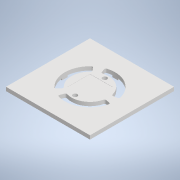
# Autodesk Inventor part: CubeFace
Saved by Autodesk Inventor 2022 (Build 260153000, 153)
## iProperties
Created: 2022-04-08
Part Number: CubeFace
Material: Generic
Document SubType Name: Modeling
Designer: awp
Density: 1 g/cm^3
Appearance: Default
Author: awp
Autodesk Inventor part; units mm, degrees
ref_plane "YZ Plane" through (0, 0, 0) normal (1, 0, 0) x (0, 1, 0)
ref_plane "XZ Plane" through (0, 0, 0) normal (0, 1, 0) x (-1, 0, 0)
ref_plane "XY Plane" through (0, 0, 0) normal (0, 0, 1) x (1, 0, 0)
sketch "Sketch1" plane through (0, 0, 0) normal (0, 1, 0) x (-1, 0, 0)
  line L0 (0, 0) -> (57.5, 0)
  line L1 (57.5, 0) -> (57.5, -57.5)
  line L2 (57.5, -57.5) -> (0, -57.5)
  line L3 (0, -57.5) -> (0, 0)
  dimension "d0" = 57.5
  dimension "d1" = 57.5
  constraints: 8 end point, 2 parallel, 1 horizontal, 1 perpendicular
  measures "d0" distance of L1.end L2.end
  measures "d1" distance of L0.end L1.end
extrude "Extrusion1" add sketch "Sketch1" along normal blind 2.54
sketch "Sketch2" plane through (0, 0, 0) normal (0, -1, 0) x (1, 0, 0)
  line L0 (0, -57.5) -> (-57.5, -57.5) projected
  line L1 (0, 0) -> (0, -57.5) projected
  line L2 (-57.5, 0) -> (0, 0) projected
  line L3 (-57.5, -57.5) -> (-57.5, 0) projected
  line L4 (-57.5, -57.5) -> (-57.5, 0) projected
  line L5 (-57.5, -57.5) -> (-38.3333, -57.5)
  line L6 (-38.3333, -57.5) -> (-38.3333, -38.3333)
  line L7 (-38.3333, -38.3333) -> (-57.5, -38.3333)
  line L8 (-57.5, -38.3333) -> (-57.5, -57.5)
  line L9 (-57.5, -38.3333) -> (-38.3333, -38.3333)
  line L10 (-38.3333, -38.3333) -> (-38.3333, -19.1667)
  line L11 (-38.3333, -19.1667) -> (-57.5, -19.1667)
  line L12 (-57.5, -19.1667) -> (-57.5, -38.3333)
  line L13 (-57.5, 0) -> (0, 0) projected
  line L14 (-57.5, -19.1667) -> (-38.3333, -19.1667)
  line L15 (-38.3333, -19.1667) -> (-38.3333, 0)
  line L16 (-38.3333, 0) -> (-57.5, 0)
  line L17 (-57.5, 0) -> (-57.5, -19.1667)
  line L18 (-38.3333, 0) -> (-19.1667, 0)
  line L19 (-19.1667, 0) -> (-19.1667, -19.1667)
  line L20 (-19.1667, -19.1667) -> (-38.3333, -19.1667)
  line L21 (-38.3333, -19.1667) -> (-38.3333, 0)
  line L22 (-19.1667, -19.1667) -> (0, -19.1667)
  line L23 (0, -19.1667) -> (0, 0)
  line L24 (0, 0) -> (-19.1667, 0)
  line L25 (-19.1667, 0) -> (-19.1667, -19.1667)
  line L26 (-19.1667, -19.1667) -> (-38.3333, -19.1667)
  line L27 (-38.3333, -19.1667) -> (-38.3333, -38.3333)
  line L28 (-38.3333, -38.3333) -> (-19.1667, -38.3333)
  line L29 (-19.1667, -38.3333) -> (-19.1667, -19.1667)
  line L30 (-19.1667, -38.3333) -> (-38.3333, -38.3333)
  line L31 (-38.3333, -38.3333) -> (-38.3333, -57.5)
  line L32 (-38.3333, -57.5) -> (-19.1667, -57.5)
  line L33 (-19.1667, -57.5) -> (-19.1667, -38.3333)
  line L34 (0, -19.1667) -> (-19.1667, -19.1667)
  line L35 (-19.1667, -19.1667) -> (-19.1667, -38.3333)
  line L36 (-19.1667, -38.3333) -> (0, -38.3333)
  line L37 (0, -38.3333) -> (0, -19.1667)
  line L38 (0, -38.3333) -> (-19.1667, -38.3333)
  line L39 (-19.1667, -38.3333) -> (-19.1667, -57.5)
  line L40 (-19.1667, -57.5) -> (0, -57.5)
  line L41 (0, -57.5) -> (0, -38.3333)
  line L42 (0, -57.5) -> (-57.5, -57.5) projected
  line L43 (-57.5, -57.5) -> (-56.23, -57.5)
  line L44 (-56.23, -57.5) -> (-56.23, -56.23)
  line L45 (-56.23, -56.23) -> (-57.5, -56.23)
  line L46 (-57.5, -56.23) -> (-57.5, -57.5)
  line L47 (-38.3333, -38.3333) -> (-52.3033, -38.3333)
  line L48 (-52.3033, -38.3333) -> (-52.3033, -52.3033)
  line L49 (-52.3033, -52.3033) -> (-38.3333, -52.3033)
  line L50 (-38.3333, -52.3033) -> (-38.3333, -38.3333)
  line L51 (-52.3033, -52.3033) -> (-56.23, -52.3033)
  line L52 (-56.23, -52.3033) -> (-56.23, -56.23)
  line L53 (-56.23, -56.23) -> (-52.3033, -56.23)
  line L54 (-52.3033, -56.23) -> (-52.3033, -52.3033)
  line L55 (-56.23, -26.7867) -> (-56.23, -30.7133)
  line L56 (-56.23, -30.7133) -> (-52.3033, -30.7133)
  line L57 (-52.3033, -26.7867) -> (-56.23, -26.7867)
  line L58 (-52.3033, -30.7133) -> (-52.3033, -26.7867)
  line L59 (-56.23, -1.27) -> (-56.23, -5.1967)
  line L60 (-56.23, -5.1967) -> (-52.3033, -5.1967)
  line L61 (-52.3033, -1.27) -> (-56.23, -1.27)
  line L62 (-52.3033, -5.1967) -> (-52.3033, -1.27)
  line L63 (-30.7133, -52.3033) -> (-30.7133, -56.23)
  line L64 (-30.7133, -56.23) -> (-26.7867, -56.23)
  line L65 (-26.7867, -52.3033) -> (-30.7133, -52.3033)
  line L66 (-26.7867, -56.23) -> (-26.7867, -52.3033)
  line L67 (-30.7133, -26.7867) -> (-30.7133, -30.7133)
  line L68 (-30.7133, -30.7133) -> (-26.7867, -30.7133)
  line L69 (-26.7867, -26.7867) -> (-30.7133, -26.7867)
  line L70 (-26.7867, -30.7133) -> (-26.7867, -26.7867)
  line L71 (-30.7133, -1.27) -> (-30.7133, -5.1967)
  line L72 (-30.7133, -5.1967) -> (-26.7867, -5.1967)
  line L73 (-26.7867, -1.27) -> (-30.7133, -1.27)
  line L74 (-26.7867, -5.1967) -> (-26.7867, -1.27)
  line L75 (-5.1967, -52.3033) -> (-5.1967, -56.23)
  line L76 (-5.1967, -56.23) -> (-1.27, -56.23)
  line L77 (-1.27, -52.3033) -> (-5.1967, -52.3033)
  line L78 (-1.27, -56.23) -> (-1.27, -52.3033)
  line L79 (-5.1967, -26.7867) -> (-5.1967, -30.7133)
  line L80 (-5.1967, -30.7133) -> (-1.27, -30.7133)
  line L81 (-1.27, -26.7867) -> (-5.1967, -26.7867)
  line L82 (-1.27, -30.7133) -> (-1.27, -26.7867)
  line L83 (-5.1967, -1.27) -> (-5.1967, -5.1967)
  line L84 (-5.1967, -5.1967) -> (-1.27, -5.1967)
  line L85 (-1.27, -1.27) -> (-5.1967, -1.27)
  line L86 (-1.27, -5.1967) -> (-1.27, -1.27)
  dimension "d5" = 19.1667
  dimension "d6" = 19.1667
  dimension "d7" = 19.1667
  dimension "d8" = 19.1667
  dimension "d9" = 1.27
  dimension "d10" = 1.27
  dimension "d11" = 13.97
  dimension "d12" = 13.97
  dimension "d15" = 25.5167
  dimension "d18" = 25.5167
  constraints: 160 end point, 24 parallel, 13 horizontal, 12 perpendicular, 2 collinear, 2 point on line, 1 vertical, 62 other
  measures "d5" distance of L5.end L6.end
  measures "d6" distance of L10.end L11.end
  measures "d7" distance of L9.end L10.end
  measures "d8" distance of L19.end L20.end
  measures "d9" distance of L45.end L44.end
  measures "d10" distance of L44.end L43.end
  measures "d11" distance of L49.end L48.end
  measures "d12" distance of L48.end L47.end
  measures "d15" distance of L51.end L55.start
  measures "d18" distance of L51.end L63.start
extrude "Extrusion2" add sketch "Sketch2" along normal blind 1.27 contours L52 L51 L54 L53 | L57 L58 L56 L55 | L61 L62 L60 L59 | L65 L66 L64 L63 | L69 L70 L68 L67 | L73 L74 L72 L71 | L77 L78 L76 L75 | L81 L82 L80 L79 | L85 L86 L84 L83
chamfer "Chamfer1" [suppressed]
sketch "Sketch3" plane through (0, 2.54, 0) normal (0, 1, 0) x (1, 0, 0)
  line L0 (0, 57.5) -> (-57.5, 57.5) projected
  line L1 (-57.5, 57.5) -> (-57.5, 0) projected
  line L2 (-57.5, 0) -> (0, 0) projected
  line L3 (0, 0) -> (0, 57.5) projected
  line L4 (-28.75, 28.75) -> (-36.37, 28.75)
  line L5 (-36.37, 28.75) -> (-36.37, 21.13)
  line L6 (-36.37, 21.13) -> (-28.75, 21.13)
  line L7 (-28.75, 21.13) -> (-28.75, 28.75)
  line L8 (-36.37, 21.13) -> (-21.13, 21.13)
  line L9 (-21.13, 21.13) -> (-21.13, 36.37)
  line L10 (-21.13, 36.37) -> (-36.37, 36.37)
  line L11 (-36.37, 36.37) -> (-36.37, 21.13)
  dimension "d26" = 7.62
  dimension "d27" = 7.62
  dimension "d30" = 15.24
  dimension "d31" = 15.24
  constraints: 16 end point, 4 parallel, 2 horizontal, 2 perpendicular
  measures "d26" distance of L6.end L5.end
  measures "d27" distance of L5.end L4.end
  measures "d30" distance of L10.end L9.end
  measures "d31" distance of L9.end L8.end
extrude "Extrusion3" cut sketch "Sketch3" against normal blind 0.127 contours L7 L6 L5 L4 | L4 L11 L10 L9 L8 L7
sketch "Sketch4" plane through (0, 0, 0) normal (0, -1, 0) x (1, 0, 0)
  line L0 (-56.23, -5.1967) -> (-56.23, -1.27) projected
  line L1 (-56.23, -1.27) -> (-52.3033, -1.27) projected
  line L2 (-52.3033, -1.27) -> (-52.3033, -5.1967) projected
  line L3 (-30.7133, -56.23) -> (-30.7133, -52.3033) projected
  line L4 (-30.7133, -52.3033) -> (-26.7867, -52.3033) projected
  line L5 (-26.7867, -52.3033) -> (-26.7867, -56.23) projected
  line L6 (-26.7867, -56.23) -> (-30.7133, -56.23) projected
  line L7 (-5.1967, -5.1967) -> (-5.1967, -1.27) projected
  line L8 (-5.1967, -1.27) -> (-1.27, -1.27) projected
  line L9 (-1.27, -1.27) -> (-1.27, -5.1967) projected
  line L10 (-1.27, -5.1967) -> (-5.1967, -5.1967) projected
  line L11 (-5.1967, -30.7133) -> (-5.1967, -26.7867) projected
  line L12 (-5.1967, -26.7867) -> (-1.27, -26.7867) projected
  line L13 (-1.27, -26.7867) -> (-1.27, -30.7133) projected
  line L14 (-1.27, -30.7133) -> (-5.1967, -30.7133) projected
  line L15 (-30.7133, -30.7133) -> (-30.7133, -26.7867) projected
  line L16 (-30.7133, -26.7867) -> (-26.7867, -26.7867) projected
  line L17 (-26.7867, -26.7867) -> (-26.7867, -30.7133) projected
  line L18 (-26.7867, -30.7133) -> (-30.7133, -30.7133) projected
  line L19 (-56.23, -30.7133) -> (-56.23, -26.7867) projected
  line L20 (-56.23, -26.7867) -> (-52.3033, -26.7867) projected
  line L21 (-52.3033, -26.7867) -> (-52.3033, -30.7133) projected
  line L22 (-52.3033, -30.7133) -> (-56.23, -30.7133) projected
  line L23 (-5.1967, -56.23) -> (-5.1967, -52.3033) projected
  line L24 (-5.1967, -52.3033) -> (-1.27, -52.3033) projected
  line L25 (-1.27, -52.3033) -> (-1.27, -56.23) projected
  line L26 (-1.27, -56.23) -> (-5.1967, -56.23) projected
  line L27 (-30.7133, -5.1967) -> (-30.7133, -1.27) projected
  line L28 (-30.7133, -1.27) -> (-26.7867, -1.27) projected
  line L29 (-26.7867, -1.27) -> (-26.7867, -5.1967) projected
  line L30 (-26.7867, -5.1967) -> (-30.7133, -5.1967) projected
  line L31 (-56.23, -52.3033) -> (-52.3033, -52.3033) projected
  line L32 (-52.3033, -52.3033) -> (-52.3033, -56.23) projected
  line L33 (-52.3033, -56.23) -> (-56.23, -56.23) projected
  line L34 (-56.23, -56.23) -> (-56.23, -52.3033) projected
  line L35 (0, -57.5) -> (-57.5, -57.5) projected
  line L36 (0, 0) -> (0, -57.5) projected
  line L37 (-57.5, 0) -> (0, 0) projected
  line L38 (-57.5, -57.5) -> (-57.5, 0) projected
  circle A0 centre (-28.75, -28.75) radius 19.7433
  circle A1 centre (-28.75, -28.75) radius 12.7
  line L39 (-28.75, -28.75) -> (-38.6217, -45.8482)
  line L40 (-28.75, -28.75) -> (-9.0067, -28.75) construction
  line L41 (-28.75, -28.75) -> (-38.6217, -11.6518)
  line L42 (-28.75, -28.75) -> (-9.0067, -28.75) construction
  line L43 (-28.75, -28.75) -> (-9.0067, -28.75)
  line L44 (-28.75, -28.75) -> (-9.0067, -28.75) construction
  line L45 (-28.75, -28.75) -> (-35.5026, -47.3027)
  line L46 (-28.75, -28.75) -> (-9.0067, -28.75) construction
  line L47 (-28.75, -28.75) -> (-41.4408, -43.8743)
  line L48 (-28.75, -28.75) -> (-9.0067, -28.75) construction
  line L49 (-28.75, -28.75) -> (-35.5026, -10.1973)
  line L50 (-28.75, -28.75) -> (-9.0067, -28.75) construction
  line L51 (-28.75, -28.75) -> (-41.4408, -13.6257)
  line L52 (-28.75, -28.75) -> (-9.0067, -28.75) construction
  line L53 (-28.75, -28.75) -> (-9.3066, -32.1784)
  line L54 (-28.75, -28.75) -> (-9.0067, -28.75) construction
  line L55 (-28.75, -28.75) -> (-9.3066, -25.3216)
  line L56 (-28.75, -28.75) -> (-9.0067, -28.75) construction
  line L57 (-52.3033, -5.1967) -> (-56.23, -5.1967) projected
  circle A2 centre (-28.75, -28.75) radius 17.2085
  line L58 (-30.7133, -26.7867) -> (-26.7867, -26.7867) projected
  line L59 (-28.75, -26.7867) -> (-28.75, -28.75)
  point P0 (-36.9134, -19.0212)
  point P1 (-36.9134, -38.4788)
  point P2 (-16.2429, -26.5447)
  point P3 (-33.0937, -16.8159)
  point P4 (-16.2429, -30.9553)
  point P5 (-33.0937, -40.6841)
  point P6 (-34.6357, -44.9207)
  point P7 (-11.8029, -31.7382)
  point P8 (-11.8029, -25.7618)
  point P9 (-34.6357, -12.5793)
  point P10 (-39.8114, -15.5675)
  point P11 (-39.8114, -41.9325)
  point P12 (-30.3974, -30.7133)
  point P13 (-30.3974, -26.7867)
  point P14 (-28.75, -52.3033)
  point P15 (-48.4933, -28.75)
  point P16 (-28.75, -9.0067)
  point P17 (-9.0067, -28.75)
  point P18 (-11.5415, -28.75)
  point P19 (-16.05, -28.75)
  point P20 (-37.3543, -43.653)
  point P21 (-37.3543, -13.847)
  point P22 (-35.1, -17.7515)
  point P23 (-26.7867, -28.4038)
  point P24 (-29.4646, -26.7867)
  point P25 (-26.7867, -29.0962)
  point P26 (-29.4646, -30.7133)
  point P27 (-29.8835, -26.7867)
  point P28 (-26.7867, -28.75)
  point P29 (-29.8835, -30.7133)
  point P30 (-35.1, -39.7485)
  dimension "d47" = 39.4867
  dimension "d32" = 25.4
  dimension "d35" = 120
  dimension "d36" = 120
  dimension "d37" = 0
  dimension "d38" = 110
  dimension "d39" = 130
  dimension "d40" = 110
  dimension "d41" = 130
  dimension "d42" = 10
  dimension "d43" = 10
  dimension "d48" = 34.417
  constraints: 38 end point, 9 equal length, 9 horizontal, 2 centre point, 2 coincident, 1 collinear, 1 midpoint, 1 vertical, 10 other
  measures "d32" diameter of A1
  measures "d35" angle of L39 L40
  measures "d36" angle of L42 L41
  measures "d37" distance between parallel lines of L43 L44
  measures "d38" angle of L45 L46
  measures "d39" angle of L47 L48
  measures "d40" angle of L50 L49
  measures "d41" angle of L52 L51
  measures "d42" angle of L53 L54
  measures "d43" angle of L56 L55
  measures "d48" diameter of A2
extrude "Extrusion4" cut sketch "Sketch4" against normal through all contours L47 A2 L51 A1 | A1 L53 A2 L45 | L49 A2 L55 A1
fillet "Fillet1" radius 0.889 12 edges at (-16.2429, 1.27, -26.5447) (-33.0937, 1.27, -16.8159) (-16.2429, 1.27, -30.9553) (-33.0937, 1.27, -40.6841) (-36.9134, 1.27, -38.4788) (-36.9134, 1.27, -19.0212) (-39.8114, 1.27, -41.9325) (-39.8114, 1.27, -15.5675) (-34.6357, 1.27, -12.5793) (-34.6357, 1.27, -44.9207) (-11.8029, 1.27, -31.7382) (-11.8029, 1.27, -25.7618)
sketch "Sketch5" plane through (0, 2.54, 0) normal (0, 1, 0) x (1, 0, 0)
  circle A0 centre (-28.7675, 18.59) radius 1.5 projected
  circle A1 centre (-28.7675, 38.875) radius 1.5 projected
  point P0 (0, 0)
extrude "Extrusion5" cut sketch "Sketch5" against normal up to surface (2.54 mm away)
thicken "Thicken1" operation add thickness 6.35 both sides no extend neighbours yes toward (0, 0, -1) faces at (-19.1667, 1.6933, -57.5) (-57.5, 1.6933, -38.3333) (-38.3333, 1.6933, 0) (0, 1.6933, -19.1667)
sketch "Sketch6" plane through (0, 2.413, 0) normal (0, 1, 0) x (1, 0, 0)
  circle A0 centre (-28.7675, 18.59) radius 1.5 projected
  circle A1 centre (-28.7675, 38.875) radius 1.5 projected
  arc A2 (-37.5324, 37.9239) -> (-37.5324, 19.5761) centre (-28.75, 28.75) ccw projected
  arc A3 (-37.4661, 18.3625) -> (-37.5324, 19.5761) centre (-38.1471, 18.934) ccw projected
  line L0 (-37.4661, 18.3625) -> (-39.2244, 16.2671) projected
  arc A4 (-40.5131, 16.1897) -> (-39.2244, 16.2671) centre (-39.9054, 16.8385) ccw projected
  arc A5 (-40.5131, 41.3103) -> (-40.5131, 16.1897) centre (-28.75, 28.75) ccw projected
  arc A6 (-39.2244, 41.2329) -> (-40.5131, 41.3103) centre (-39.9054, 40.6615) ccw projected
  line L1 (-39.2244, 41.2329) -> (-37.4661, 39.1375) projected
  arc A7 (-37.5324, 37.9239) -> (-37.4661, 39.1375) centre (-38.1471, 38.566) ccw projected
  arc A8 (-32.3036, 16.5573) -> (-16.414, 25.7312) centre (-28.75, 28.75) ccw projected
  arc A9 (-15.3961, 26.3953) -> (-16.414, 25.7312) centre (-15.5505, 25.5199) ccw projected
  line L2 (-15.3961, 26.3953) -> (-12.7023, 25.9204) projected
  arc A10 (-11.9909, 24.843) -> (-12.7023, 25.9204) centre (-12.8567, 25.0449) ccw projected
  arc A11 (-33.746, 12.2827) -> (-11.9909, 24.843) centre (-28.75, 28.75) ccw projected
  arc A12 (-34.3233, 13.4375) -> (-33.746, 12.2827) centre (-33.4879, 13.1334) ccw projected
  line L3 (-34.3233, 13.4375) -> (-33.3878, 16.0079) projected
  arc A13 (-32.3036, 16.5573) -> (-33.3878, 16.0079) centre (-32.5524, 15.7038) ccw projected
  arc A14 (-16.414, 31.7688) -> (-32.3036, 40.9427) centre (-28.75, 28.75) ccw projected
  arc A15 (-33.3878, 41.4921) -> (-32.3036, 40.9427) centre (-32.5524, 41.7962) ccw projected
  line L4 (-33.3878, 41.4921) -> (-34.3233, 44.0625) projected
  arc A16 (-33.746, 45.2173) -> (-34.3233, 44.0625) centre (-33.4879, 44.3666) ccw projected
  arc A17 (-11.9909, 32.657) -> (-33.746, 45.2173) centre (-28.75, 28.75) ccw projected
  arc A18 (-12.7023, 31.5796) -> (-11.9909, 32.657) centre (-12.8567, 32.4551) ccw projected
  line L5 (-12.7023, 31.5796) -> (-15.3961, 31.1047) projected
  arc A19 (-16.414, 31.7688) -> (-15.3961, 31.1047) centre (-15.5505, 31.9801) ccw projected
  line L6 (-21.13, 21.13) -> (-36.37, 21.13) projected
  line L7 (-36.37, 21.13) -> (-36.37, 36.37) projected
  line L8 (-36.37, 36.37) -> (-21.13, 36.37) projected
  line L9 (-21.13, 36.37) -> (-21.13, 21.13) projected
  line L10 (6.35, 63.85) -> (-63.85, 63.85) projected
  line L11 (-63.85, 63.85) -> (-63.85, -6.35) projected
  line L12 (-63.85, -6.35) -> (6.35, -6.35) projected
  line L13 (6.35, -6.35) -> (6.35, 63.85) projected
  line L14 (-36.37, 21.13) -> (-36.37, 36.37) projected
  line L15 (-21.13, 21.13) -> (-36.37, 21.13) projected
  line L16 (-21.13, 36.37) -> (-21.13, 21.13) projected
  line L17 (-36.37, 36.37) -> (-21.13, 36.37) projected
  line L18 (-24, 33.5) -> (-33.5, 33.5)
  line L19 (-33.5, 33.5) -> (-33.5, 24)
  line L20 (-33.5, 24) -> (-24, 24)
  line L21 (-24, 24) -> (-24, 33.5)
  line L22 (-24, 33.5) -> (-33.5, 24) construction
  line L23 (-33.5, 33.5) -> (-24, 24) construction
  line L24 (-28.75, 28.75) -> (-31.29, 28.75)
  line L25 (-28.75, 28.75) -> (-26.21, 28.75)
  line L26 (-28.75, 28.75) -> (-26.21, 28.75) construction
  line L27 (-28.75, 28.75) -> (-28.75, 31.29)
  line L28 (-28.75, 28.75) -> (-26.21, 28.75) construction
  circle A20 centre (-31.29, 28.75) radius 0.635
  circle A21 centre (-28.75, 31.29) radius 0.635
  circle A22 centre (-26.21, 28.75) radius 0.635
  point P0 (0, 0)
  dimension "d51" = 9.5
  dimension "d52" = 9.5
  dimension "d53" = 2.54
  dimension "d54" = 2.54
  dimension "d55" = 0
  dimension "d56" = 2.54
  dimension "d57" = 90
  dimension "d58" = 1.27
  dimension "d59" = 1.27
  dimension "d60" = 1.27
  constraints: 22 end point, 5 horizontal, 3 centre point, 3 coincident, 2 equal length, 2 midpoint, 2 parallel, 2 perpendicular
  measures "d51" distance of L18.start L18.end
  measures "d52" distance of L19.end L18.end
  measures "d53" distance of L24.start L24.end
  measures "d54" distance of L24.start L25.end
  measures "d55" distance between parallel lines of L25 L26
  measures "d56" distance of L24.start L27.end
  measures "d57" angle of L28 L27
  measures "d58" diameter of A20
  measures "d59" diameter of A21
  measures "d60" diameter of A22
extrude "Extrusion6" cut sketch "Sketch6" against normal blind 25.4 contours A20 | A21 | A22
equation "\"d5\" = d4"
equation "\"d6\" = d4"
equation "\"d7\" = d4"
equation "\"d8\" = d4"
equation "\"d4\" = 19.166667"
body "Solid1"
